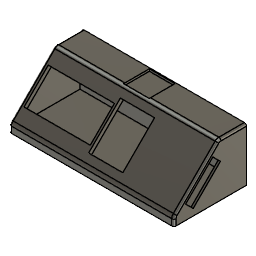
timer (Autodesk Fusion 360 design; units mm, degrees)
Autodesk Fusion 360 part; units mm, degrees
sketch "Sketch1" plane through (0, 0, 0) normal (0, 0, 1) x (1, 0, 0)
  line L0 (-90, 100) -> (-60, 100)
  line L1 (-60, 100) -> (-60, 85)
  line L2 (-60, 85) -> (-90, 85)
  line L3 (-90, 85) -> (-90, 100)
  line L4 (-47.5674, 100) -> (-32.5674, 100)
  line L5 (-32.5674, 100) -> (-32.5674, 80)
  line L6 (-32.5674, 80) -> (-47.5674, 80)
  line L7 (-47.5674, 80) -> (-47.5674, 100)
  line L8 (25, 15) -> (-25, 15)
  line L9 (-25, 15) -> (-25, -15)
  line L10 (-25, -15) -> (25, -15)
  line L11 (25, -15) -> (25, 15)
  line L12 (25, 15) -> (-25, -15) construction
  line L13 (-25, 15) -> (25, -15) construction
  dimension "d1" = 30
  dimension "d2" = 15
  dimension "d3" = 15
  dimension "d4" = 20
  dimension "d5" = 50
  dimension "d6" = 30
  constraint horizontal L0
  constraint vertical L1
  constraint horizontal L2
  constraint vertical L3
  constraint horizontal L4
  constraint vertical L5
  constraint horizontal L6
  constraint vertical L7
  constraint horizontal L8
  constraint perpendicular L8 L9
  constraint parallel L8 L10
  constraint parallel L9 L11
  constraint coincident L12 origin
  constraint coincident L13 origin
  measures "d1" distance of L0.start L0.end
  measures "d2" distance of L0.start L2.end
  measures "d3" distance of L4.start L4.end
  measures "d4" distance of L4.start L6.end
  measures "d5" distance of L9.end L10.end
  measures "d6" distance of L8.end L9.end
extrude "Extrude1" add sketch "Sketch1" along normal blind 25 contours L8 L9 L10 L11 makes body 1
chamfer "Chamfer1" distance 21 angle 45 1 edges at (0, -15, 25) on bodies 1
sketch "Sketch2" plane through (25, 0, 0) normal (1, 0, 0) x (0, 1, 0)
  line L0 (6, 25) -> (-15, 4)
  line L1 (-15, 4) -> (-15, 0)
  line L2 (-15, 0) -> (15, 0)
  line L3 (15, 25) -> (6, 25)
  line L4 (15, 25) -> (6, 25)
  line L5 (6, 25) -> (-15, 4)
  line L6 (-15, 4) -> (-15, 0)
  line L7 (-15, 0) -> (15, 0)
  line L8 (15, 25) -> (19, 25)
  line L9 (19, 25) -> (19, 0)
  line L10 (19, 0) -> (15, 0)
  dimension "d50" = 4
  constraint coincident L3.start L4.start
  constraint coincident L0.start L3.end
  constraint coincident L0.end L1.start
  constraint coincident L1.end L2.start
  constraint coincident L2.end L7.end
  constraint perpendicular L3 L9
  measures "d50" distance of L3.start L8.end
extrude "Extrude2" add sketch "Sketch2" against normal blind 75 thin wall 2 inside separate body makes body 2
extrude "Extrude3" add sketch "Sketch2" along normal blind 1 from surface at -76 bodies 2
extrude "Extrude4" add sketch "Sketch2" along normal blind 1 separate body makes body 3
sketch "Sketch3" plane through (0, -9.5, 9.5) normal (0, -0.707107, 0.707107) x (1, 0, 0)
  line L0 (25, -7.7782) -> (25, 21.9203)
  line L1 (25, 21.9203) -> (-51, 21.9203)
  line L2 (-51, -7.7782) -> (25, -7.7782)
  line L3 (-48.5, 14.5713) -> (-18.5, 14.5713)
  line L4 (-18.5, 14.5713) -> (-18.5, -0.4287)
  line L5 (-18.5, -0.4287) -> (-48.5, -0.4287)
  line L6 (-48.5, -0.4287) -> (-48.5, 14.5713)
  line L7 (-16.5, 17.0713) -> (-1.5, 17.0713)
  line L8 (-1.5, 17.0713) -> (-1.5, -2.9287)
  line L9 (-1.5, -2.9287) -> (-16.5, -2.9287)
  line L10 (-16.5, -2.9287) -> (-16.5, 17.0713)
  line L11 (-18, 15.0713) -> (-49, 15.0713)
  line L12 (-49, 15.0713) -> (-49, -0.9287)
  line L13 (-49, -0.9287) -> (-18, -0.9287)
  line L14 (-18, -0.9287) -> (-18, 15.0713)
  line L15 (-18, 15.0713) -> (-49, -0.9287) construction
  line L16 (-49, 15.0713) -> (-18, -0.9287) construction
  line L17 (-1, 17.5713) -> (-17, 17.5713)
  line L18 (-17, 17.5713) -> (-17, -3.4287)
  line L19 (-17, -3.4287) -> (-1, -3.4287)
  line L20 (-1, -3.4287) -> (-1, 17.5713)
  line L21 (-1, 17.5713) -> (-17, -3.4287) construction
  line L22 (-17, 17.5713) -> (-1, -3.4287) construction
  line L23 (-51, 21.9203) -> (-51, -7.7782)
  line L24 (0, 17.0713) -> (25, 17.0713)
  line L25 (25, 17.0713) -> (25, -2.9287)
  line L26 (25, -2.9287) -> (0, -2.9287)
  line L27 (0, -2.9287) -> (0, 17.0713)
  point P0 (-33.5, 7.0713)
  point P1 (-9, 7.0713)
  dimension "d18" = 30
  dimension "d19" = 15
  dimension "d20" = 15
  dimension "d21" = 20
  dimension "d22" = 7.349
  dimension "d23" = 4.849
  dimension "d24" = 31
  dimension "d25" = 16
  dimension "d26" = 16
  dimension "d27" = 21
  dimension "d28" = 1
  dimension "d30" = 0.5
  dimension "d31" = 0.5
  dimension "d32" = 0.5
  dimension "d33" = 0.5
  dimension "d34" = 2
  dimension "d35" = 25
  dimension "d36" = 20
  dimension "d37" = 1
  dimension "d38" = 4.849
  constraint horizontal L3
  constraint vertical L4
  constraint horizontal L5
  constraint vertical L6
  constraint horizontal L7
  constraint vertical L8
  constraint horizontal L9
  constraint vertical L10
  constraint horizontal L11
  constraint perpendicular L11 L12
  constraint parallel L11 L13
  constraint parallel L12 L14
  constraint coincident L15 P0
  constraint coincident L16 P0
  constraint horizontal L17
  constraint perpendicular L17 L18
  constraint parallel L17 L19
  constraint parallel L18 L20
  constraint coincident L21 P1
  constraint coincident L22 P1
  constraint horizontal L24
  constraint vertical L25
  constraint horizontal L26
  constraint vertical L27
  measures "d18" distance of L3.start L3.end
  measures "d19" distance of L3.start L5.end
  measures "d20" distance of L7.start L7.end
  measures "d21" distance of L7.start L9.end
  measures "d22" distance of L1 L3
  measures "d23" distance of L1 L7
  measures "d24" distance of L12.end L13.end
  measures "d25" distance of L11.end L12.end
  measures "d26" distance of L18.end L19.end
  measures "d27" distance of L17.end L18.end
  measures "d28" distance of L14 L18
  measures "d30" distance of L3 L11
  measures "d31" distance of L4 L14
  measures "d32" distance of L10 L18
  measures "d33" distance of L9 L19
  measures "d34" distance of L12 L23
  measures "d35" distance of L24.start L24.end
  measures "d36" distance of L24.start L26.end
  measures "d37" distance of L20 L27
  measures "d38" distance of L1 L24
sketch "Sketch4" plane through (26, 0, 0) normal (1, 0, 0) x (0, 1, 0)
  line L0 (19, 25) -> (6, 25)
  line L1 (6, 25) -> (-15, 4)
  line L2 (-15, 4) -> (-15, 0)
  line L3 (-15, 0) -> (19, 0)
  line L4 (-9.5217, 6.6499) -> (3.2062, 19.3778)
  line L5 (3.2062, 19.3778) -> (6.7418, 15.8423)
  line L6 (6.7418, 15.8423) -> (-5.9862, 3.1143)
  line L7 (-9.5217, 6.6499) -> (-5.9862, 3.1143)
  line L8 (19, 0) -> (19, 25)
  point P0 (-11.5709, 7.4291)
  point P1 (2.5712, 21.5712)
  dimension "d39" = 18
  dimension "d40" = 5
  dimension "d41" = 18
  dimension "d44" = 2
  dimension "d47" = 2.2835
  constraint parallel L1 L4
  constraint perpendicular L4 L5
  constraint perpendicular L5 L6
  measures "d39" distance of L4.start L4.end
  measures "d40" distance of L4.end L5.end
  measures "d41" distance of L5.end L6.end
  measures "d44" distance of L1 L4
  measures "d47" distance of L4.end P1
extrude "Extrude5" cut sketch "Sketch4" against normal blind 2 contours L4 L5 L6 L7 bodies 2 3
sketch "Sketch5" plane through (0, 0, 25) normal (0, 0, 1) x (-1, 0, 0)
  line L0 (-25, -6) -> (-25, -19)
  line L1 (51, -19) -> (51, -6)
  line L2 (51, -6) -> (-25, -6)
  line L3 (19, -18.5) -> (7, -18.5)
  line L4 (7, -18.5) -> (7, -6.5)
  line L5 (7, -6.5) -> (19, -6.5)
  line L6 (19, -6.5) -> (19, -18.5)
  line L7 (-25, -19) -> (51, -19)
  dimension "d48" = 12
  dimension "d49" = 12
  dimension "d51" = 0.5
  dimension "d52" = 32
  constraint horizontal L3
  constraint vertical L4
  constraint horizontal L5
  constraint vertical L6
  measures "d48" distance of L3.start L3.end
  measures "d49" distance of L3.start L5.end
  measures "d51" distance of L3 L7
  measures "d52" distance of L0 L4
sketch "Sketch6" plane through (26, 0, 0) normal (1, 0, 0) x (0, 1, 0)
  line L0 (-5.9862, 3.1143) -> (-9.5217, 6.6499)
  line L1 (-9.5217, 6.6499) -> (3.2062, 19.3778)
  line L2 (3.2062, 19.3778) -> (6.7418, 15.8423)
  line L3 (6.7418, 15.8423) -> (-5.9862, 3.1143)
  line L4 (19, 25) -> (6, 25)
  line L5 (6, 25) -> (-15, 4)
  line L6 (-15, 4) -> (-15, 0)
  line L7 (-15, 0) -> (19, 0)
  line L8 (19, 0) -> (19, 25)
fillet "Fillet1" radius 2.5 1 edges at (-13, -15, 4) on bodies 2
fillet "Fillet2" radius 2.5 1 edges at (-13, 6, 25) on bodies 2
fillet "Fillet3" radius 2.5 2 edges at (25.5, 6, 25) (25.5, -15, 4) on bodies 3
fillet "Fillet4" radius 1 10 edges at (-51, 13.0178, 25) (-51, 6.0788, 24.8097) (-51, -4.5, 14.5) (-51, -14.8097, 3.9212) (-51, -15, 1.4822) (26, 13.0178, 25) (26, 6.0788, 24.8097) (26, -4.5, 14.5) (26, -14.8097, 3.9212) (26, -15, 1.4822) on bodies 2 3
move_body "Move1" bodies 3 to x (1, 0, 0) y (0, 1, 0) z (0, 0, 1) at (0, -35, 0)
sketch "Sketch7" plane through (0, 0, 2) normal (0, 0, 1) x (-1, 0, 0)
  line L0 (-25, 13) -> (-25, -17)
  line L1 (-25, -17) -> (50, -17)
  line L2 (50, -17) -> (50, 13)
  line L3 (50, 13) -> (-25, 13)
  line L4 (-25, -17) -> (-28, -17)
  line L5 (-28, -17) -> (-28, -14)
  line L6 (-28, -14) -> (-25, -14)
  line L7 (-25, -14) -> (-25, -17)
  line L8 (-25, -17) -> (-22, -17)
  line L9 (-22, -17) -> (-22, -14)
  line L10 (-22, -14) -> (-25, -14)
  line L11 (-25, -14) -> (-25, -17)
  circle A0 centre (-29.75, -15.705) radius 1.75
  line L12 (-28, -17) -> (-28.5729, -17)
  line L13 (-28, -14) -> (-29.3557, -14)
  circle A1 centre (-29.75, -15.705) radius 1.5
  line L14 (-29.75, -14.205) -> (-35.75, -14.205)
  line L15 (-35.75, -14.205) -> (-35.75, -17.2525)
  line L16 (-35.75, -17.2525) -> (-29.7381, -17.2049)
  dimension "d61" = 3
  dimension "d62" = 3
  dimension "d63" = 3.5
  dimension "d64" = 3
  dimension "d65" = 6
  constraint horizontal L4
  constraint vertical L5
  constraint horizontal L6
  constraint vertical L7
  constraint coincident L0.end L1.start
  constraint horizontal L8
  constraint vertical L9
  constraint horizontal L10
  constraint vertical L11
  constraint coincident A0 L12.end
  constraint perpendicular L5 L12
  constraint coincident A0 L13.end
  constraint perpendicular L5 L13
  constraint tangent L5 A0
  constraint concentric A0 A1
  constraint coincident A1 L14.start
  constraint parallel L13 L14
  constraint perpendicular L14 L15
  constraint coincident A1 L16.end
  constraint tangent A1 L16
  constraint tangent A1 L14
  measures "d61" distance of L0.end L4.end
  measures "d62" distance of L0.end L6.end
  measures "d63" diameter of A0
  measures "d64" diameter of A1
  measures "d65" distance of L14.start L14.end
extrude "Extrude6" add sketch "Sketch7" along normal blind 4.5 separate body contours A0 A1 L14 L16 | A0 A1 L14 L16 makes body 4
extrude "Extrude7" add sketch "Sketch7" along normal blind 6.3 separate body contours A1 makes body 5
extrude "Extrude8" add sketch "Sketch7" along normal blind 1.5 from surface at 4.8 contours A0 A1 L14 L16 | A0 L14 L15 L16 picked at (-31.4084, -15.8348) bodies 5
extrude "Extrude9" add sketch "Sketch7" along normal blind 1.5 contours L0 L1 L7 L8 L9 L10 L11 | L0 L4 L5 L6 L7 L11 | L5 A0 L13 | L5 A0 L12 bodies 4
move_body "Move2" bodies 4 5 to x (1, 0, 0) y (0, 1, 0) z (0, 0, 1) at (8, 0, 0)
move_body "Move4" bodies 5 4 to x (1, 0, 0) y (0, 1, 0) z (0, 0, 1) at (-15.5, 0, 0)
move_body "Move6" bodies 4 5 to x (1, 0, 0) y (0, 1, 0) z (0, 0, 1) at (1, 0, 0)
copy_body "Body->Comp2" bodies 5 removing the originals makes body 6 in component "Component"
copy_body "Body->Comp4" bodies 4 removing the originals makes body 7 in component "Component'"
copy_body "CopyPasteBodies2" bodies 6 7 makes body 8 makes body 9
move_body "Move7" bodies 8 9 to x (1, 0, 0) y (0, 1, 0) z (0, 0, 1) at (0, 0, 13)
move_body "Move8" bodies 8 to x (0, -1, 0) y (1, 0, 0) z (0, 0, 1) at (7.545, 38.955, 0)
move_body "Move9" bodies 3 to x (1, 0, 0) y (0, 1, 0) z (0, 0, 1) at (0, 35, 0)
extrude "Extrude10" cut sketch "Sketch3" against normal blind 2 contours L3 L4 L5 L6 | L7 L8 L9 L10 | L11 L12 L13 L14 | L17 L18 L19 L20 bodies 2
extrude "Extrude11" cut sketch "Sketch5" against normal blind 1 contours L3 L4 L5 L6 bodies 2
component "Component" placed x (0, -1, 0) y (1, 0, 0) z (0, 0, 1) at (7.545, 38.955, 0)
component "Component'" placed x (1, 0, 0) y (0, 1, 0) z (0, 0, 1) at (0, 0, 0)
hidden bodies 1
